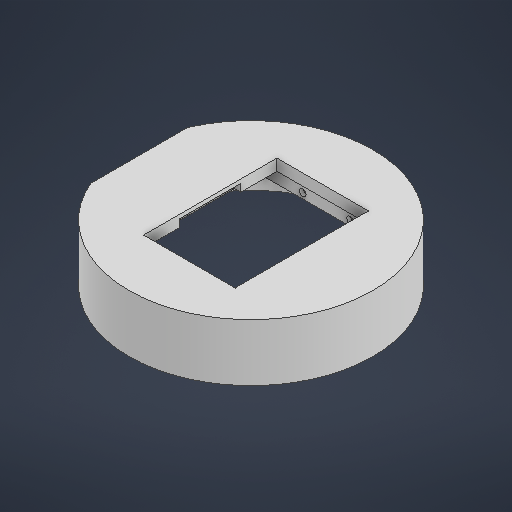
# Autodesk Inventor part: Deckel
Saved by Autodesk Inventor 2026 (Build 300175000, 175)
## iProperties
Created: 2025-04-30
Part Number: Deckel
Material: Generisch
Document SubType Name: Modeling
Designer: HTL
Density: 1 g/cm^3
Appearance: Vorgabe
Author: HTL
Autodesk Inventor part; units mm, degrees
ref_plane "YZ Plane" through (0, 0, 0) normal (1, 0, 0) x (0, 1, 0)
ref_plane "XZ Plane" through (0, 0, 0) normal (0, 1, 0) x (-1, 0, 0)
ref_plane "XY Plane" through (0, 0, 0) normal (0, 0, 1) x (1, 0, 0)
sketch "Skizze1" plane through (0, 0, 0) normal (0, 0, 1) x (1, 0, 0)
  arc A0 (-28.686, -12.2792) -> (-28.686, 12.2792) centre (-1.314, 0) ccw projected
  line L0 (-28.686, -12.2792) -> (-28.686, 12.2792) projected
  line L1 (-29.486, 12.4492) -> (-29.486, -12.4492) projected
  arc A1 (-29.486, -12.4492) -> (-29.486, 12.4492) centre (-1.314, 0) ccw projected
  arc A2 (-30.686, -12.7) -> (-30.686, 12.7) centre (-1.314, 0) ccw projected
  line L2 (-30.686, 12.7) -> (-30.686, -12.7) projected
  point P0 (0, 0)
extrude "Extrusion1" add sketch "Skizze1" against normal blind 4 contours L2 A2
sketch "Skizze2" plane through (0, 0, 0) normal (0, 0, 1) x (1, 0, 0)
  line L0 (-30.686, 12.7) -> (-30.686, -12.7) projected
  arc A0 (-30.686, -12.7) -> (-30.686, 12.7) centre (-1.314, 0) ccw projected
  arc A1 (-28.686, -12.2792) -> (-28.686, 12.2792) centre (-1.314, 0) ccw projected
  line L1 (-28.686, -12.2792) -> (-28.686, 12.2792) projected
  point P0 (0, 0)
extrude "Extrusion2" add sketch "Skizze2" along normal blind 8
sketch "Skizze3" plane through (0, 0, 8) normal (0, 0, 1) x (1, 0, 0)
  arc A0 (-30.686, -12.7) -> (-30.686, 12.7) centre (-1.314, 0) ccw projected
  line L0 (-30.686, 12.7) -> (-30.686, -12.7) projected
  point P0 (0, 0)
extrude "Extrusion3" add sketch "Skizze3" along normal blind 2
sketch "Skizze4" plane through (0, 0, 10) normal (0, 0, 1) x (1, 0, 0)
  line L0 (12, -17.5) -> (-12, -17.5)
  line L1 (-12, 17.5) -> (12, 17.5)
  line L2 (-17.2, 8) -> (-17.2, -8)
  line L3 (-17.2, -8) -> (-12, -8)
  line L4 (-12, 8) -> (-17.2, 8)
  line L5 (-12, -17.5) -> (-12, -8)
  line L6 (-12, 8) -> (-12, 17.5)
  line L7 (17.2, -8) -> (17.2, 8)
  line L8 (-17.2, 8) -> (-17.2, -8)
  line L9 (-17.2, -8) -> (-12, -8)
  line L10 (12, -8) -> (17.2, -8)
  line L11 (17.2, 8) -> (12, 8)
  line L12 (-12, 8) -> (-17.2, 8)
  line L13 (12, 17.5) -> (12, 8)
  line L14 (12, -8) -> (12, -17.5)
  point P0 (0, 0)
  dimension "d32" = 34.4
  constraints: 30 end point, 11 parallel, 5 perpendicular, 2 horizontal
  measures "d32" distance of L8.start L7.end
extrude "Extrusion4" cut sketch "Skizze4" against normal blind 2
sketch "Skizze5" plane through (0, 0, 8) normal (0, 0, -1) x (-1, 0, 0)
  line L0 (17, 18) -> (-17, -18) construction
  line L1 (17, -18) -> (-17, 18) construction
  line L2 (-17.5, -18.5) -> (17.5, -18.5)
  line L3 (17.5, -18.5) -> (17.5, 18.5)
  line L4 (17.5, 18.5) -> (-17.5, 18.5)
  line L5 (-17.5, 18.5) -> (-17.5, -18.5)
  line L6 (18.5, -19.5) -> (-18.5, -19.5)
  line L7 (-18.5, -19.5) -> (-18.5, 19.5)
  line L8 (-18.5, 19.5) -> (18.5, 19.5)
  line L9 (18.5, 19.5) -> (18.5, -19.5)
  point P0 (0, 0)
  dimension "d17" = 1
  constraints: 20 end point, 4 parallel, 2 midpoint, 2 perpendicular, 3 other
  measures "d17" distance between parallel lines of L2 L6
extrude "Extrusion5" add sketch "Skizze5" along normal blind 3.9
sketch "Skizze7" plane through (-18.5, 19.5, 8) normal (0, 1, 0) x (1, 0, 0)
  line L0 (0, 0) -> (0, 3.9) projected
  line L1 (37, 0) -> (37, 3.9) projected
  line L2 (0, 0) -> (37, 0)
  line L3 (37, 0) -> (37, 2.475)
  line L4 (0, 2.475) -> (0, 0)
  circle A0 centre (24.7, 2.475) radius 0.875
  circle A1 centre (12.3, 2.475) radius 0.875
  point P0 (18.5, 8)
  dimension "d25" = 2.475
  dimension "d28" = 1.75
  dimension "d29" = 1.75
  constraints: 6 end point, 2 centre point, 1 horizontal, 1 parallel, 1 perpendicular, 1 point on line
  measures "d25" distance of L3.end L2.end
  measures "d28" diameter of A0
  measures "d29" diameter of A1
extrude "Extrusion6" cut sketch "Skizze7" against normal blind 40
sketch "Skizze8" plane through (0, 0, 10) normal (0, 0, 1) x (1, 0, 0)
  arc A0 (-30.686, -12.7) -> (-30.686, 12.7) centre (-1.314, 0) ccw projected
  line L0 (-30.686, 12.7) -> (-30.686, -12.7) projected
  line L1 (-12, 8) -> (-12, 17.5) projected
  line L2 (12, -17.5) -> (12, -8) projected
  line L3 (-12, 17.5) -> (12, 17.5)
  line L4 (12, 17.5) -> (12, -17.5)
  line L5 (12, -17.5) -> (-12, -17.5)
  line L6 (-12, -17.5) -> (-12, 17.5)
  point P0 (0, 0)
  constraints: 8 end point, 2 parallel, 1 horizontal, 1 perpendicular
extrude "Extrusion7" add sketch "Skizze8" along normal blind 1
